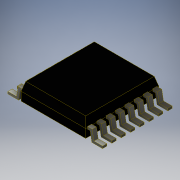
# Autodesk Inventor part: TSSOP-16
Saved by Autodesk Inventor 2016 (Build 200138000, 138)
## iProperties
Created: 2016-09-14
Part Number: TSSOP-16
Material: Generic
Document SubType Name: Modeling
Designer: jfixelle
Density: 1 g/cm^3
Appearance: Silver
Author: jfixelle
Autodesk Inventor part; units mm, degrees
ref_plane "YZ Plane" through (0, 0, 0) normal (1, 0, 0) x (0, 1, 0)
ref_plane "XZ Plane" through (0, 0, 0) normal (0, 1, 0) x (-1, 0, 0)
sketch "Sketch1" plane through (0, 0, 0) normal (0, 1, 0) x (-1, 0, 0)
  line L0 (2.25, 2.55) -> (-2.25, 2.55)
  line L1 (-2.25, 2.55) -> (-2.25, -2.55)
  line L2 (-2.25, -2.55) -> (2.25, -2.55)
  line L3 (2.25, -2.55) -> (2.25, 2.55)
  point P0 (0, 0)
  dimension "d0" = 5.1
  dimension "d1" = 2.55
  dimension "d2" = 4.5
  dimension "d3" = 2.25
  constraints: 8 end point, 2 parallel, 1 horizontal, 1 perpendicular
  measures "d0" distance of L2.end L0.start
  measures "d1" distance from line of point (0, 0) L2
  measures "d2" distance of L1.end L2.end
  measures "d3" distance from line of point (0, 0) L3
extrude "Extrusion1" add sketch "Sketch1" along normal blind 1.2
ref_plane "Work Plane1" through (0, 0, 0.325) normal (0, 0, 1) x (1, 0, 0)
chamfer "Chamfer1" distance 0.6 angle 15 1 edges at (2.25, 1.2, 0) measured on face at (2.25, 0.4, 0.85)
chamfer "Chamfer2" distance 0.6 angle 15 1 edges at (-0.0804, 1.2, 2.55) measured on face at (-0.8036, 0.8, 2.55)
chamfer "Chamfer3" distance 0.6 angle 15 1 edges at (-0.0804, 1.2, -2.55) measured on face at (-0.8036, 0.8, -2.55)
chamfer "Chamfer4" distance 0.6 angle 15 1 edges at (-2.25, 1.2, 0) measured on face at (-2.25, 0.4, -0.7964)
sketch "Sketch2" plane through (0, 0, 0.325) normal (0, 0, 1) x (1, 0, 0)
  line L0 (-2.5799, 0.65) -> (-1.9432, 0.65)
  line L1 (-1.9432, 0.65) -> (-1.9432, 0.5)
  line L2 (-1.9432, 0.5) -> (-2.4354, 0.5)
  line L3 (-2.4354, 0.5) -> (-2.55, -0.15)
  line L4 (-2.55, -0.15) -> (-3.3, -0.15)
  line L5 (-3.3, -0.15) -> (-3.3, 0)
  line L6 (-3.3, 0) -> (-2.6945, 0)
  line L7 (-2.6945, 0) -> (-2.5799, 0.65)
  line L8 (2.25, 0) -> (-2.25, 0) projected
  line L9 (0, 0) -> (0, -0.1894)
  dimension "d19" = 0.15
  dimension "d20" = 0.15
  dimension "d21" = 0.15
  dimension "d22" = 3.3
  dimension "d23" = 0.65
  dimension "d24" = 0.75
  dimension "d25" = 80
  dimension "d26" = 80
  constraints: 18 end point, 4 perpendicular, 1 horizontal, 1 parallel, 1 vertical
  measures "d19" distance between parallel lines of L8 L4
  measures "d20" distance of L4.end L5.end
  measures "d21" distance between parallel lines of L2 L0
  measures "d22" distance between parallel lines of L5 L9
  measures "d23" distance between parallel lines of L8 L0
  measures "d24" distance of L3.end L4.end
  measures "d25" angle of L4 L3
  measures "d26" angle of L6 L7
extrude "Extrusion2" add sketch "Sketch2" along normal mid plane 0.3
pattern_linear "Rectangular Pattern1" count 8 spacing 0.65 along (0, 0, -1) of "Extrusion2" first direction both ways yes
mirror "Mirror1" about plane through (0, 0, 0) normal (1, 0, 0) of "Extrusion2", "Rectangular Pattern1"
body "Solid1"
